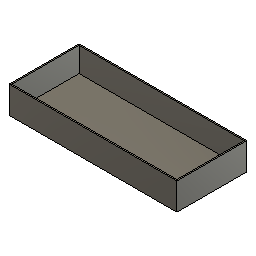
Kasten (Autodesk Fusion 360 design; units mm, degrees)
Autodesk Fusion 360 part; units mm, degrees
sketch "Sketch1" plane through (0, 0, 0) normal (0, 1, 0) x (1, 0, 0)
  line L0 (48, 20) -> (-48, 20)
  line L1 (-48, 20) -> (-48, -20)
  line L2 (-48, -20) -> (48, -20)
  line L3 (48, -20) -> (48, 20)
  line L4 (48, 20) -> (-48, -20) construction
  line L5 (-48, 20) -> (48, -20) construction
  line L6 (47.25, 19.25) -> (-47.25, 19.25)
  line L7 (-47.25, 19.25) -> (-47.25, -19.25)
  line L8 (-47.25, -19.25) -> (47.25, -19.25)
  line L9 (47.25, -19.25) -> (47.25, 19.25)
  line L10 (47.25, 19.25) -> (-47.25, -19.25) construction
  line L11 (-47.25, 19.25) -> (47.25, -19.25) construction
  dimension "d1" = 96
  dimension "d2" = 40
  dimension "d3" = 94.5
  dimension "d4" = 38.5
extrude "Extrude1" add sketch "Sketch1" along normal blind 14
sketch "Sketch2" plane through (0, 0, 0) normal (0, 1, 0) x (1, 0, 0)
  line L0 (-48, -20) -> (48, -20)
  line L1 (48, -20) -> (48, 20)
  line L2 (48, 20) -> (-48, 20)
  line L3 (-48, 20) -> (-48, -20)
extrude "Extrude2" add sketch "Sketch2" against normal blind 1.5
sketch "Sketch3" plane through (0, -1.5, 0) normal (0, -1, 0) x (1, 0, 0)
  line L0 (-48, 20) -> (-48, -20)
  line L1 (-48, -20) -> (48, -20)
  line L2 (48, -20) -> (48, 20)
  line L3 (48, 20) -> (-48, 20)
  circle A0 centre (-40.3833, 13.3405) radius 2.5
  dimension "d10" = 5
  measures "d10" diameter of A0
extrude "Extrude3" cut sketch "Sketch3" against normal blind 2.918 contours A0
